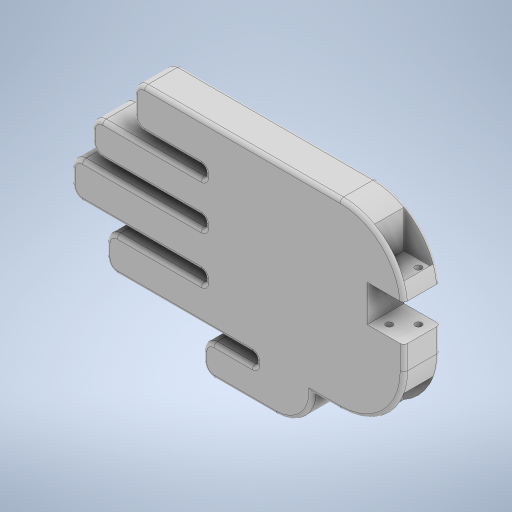
# Autodesk Inventor part: Handv3
Saved by Autodesk Inventor 2024 (Build 280153000, 153)
## iProperties
Created: 2024-02-01
Part Number: Handv3
Material: Generic
Document SubType Name: Modeling
Designer: Irwin
Density: 1 g/cm^3
Appearance: Default
Author: Irwin
Autodesk Inventor part; units mm, degrees
ref_plane "XY Plane" through (0, 0, 0) normal (0, 0, 1) x (1, 0, 0)
sketch "Sketch1" plane through (0, 0, 0) normal (0, 0, 1) x (1, 0, 0)
  line L0 (0, 0) -> (-95, 0)
  line L1 (-95, 0) -> (-95, 100)
  line L2 (-95, 100) -> (0, 100)
  line L3 (0, 100) -> (0, 0)
  dimension "d0" = 100
  dimension "d1" = 95
  constraints: 8 end point, 2 parallel, 1 horizontal, 1 perpendicular
  measures "d0" distance of L2.end L0.start
  measures "d1" distance of L0.start L0.end
extrude "Extrusion1" add sketch "Sketch1" against normal blind 20
sketch "Sketch2" plane through (-95, 0, 0) normal (-1, 0, 0) x (0, 0, 1)
  circle A0 centre (-10, 10) radius 10
  circle A1 centre (-10, 37) radius 10
  circle A2 centre (-10, 63) radius 10
  circle A3 centre (-10, 90) radius 10
  line L0 (0, 0) -> (-20, 0) projected
  line L1 (0, 100) -> (-20, 100) projected
  line L2 (-20, 0) -> (-20, 100) projected
  line L3 (0, 0) -> (-20, 0)
  line L4 (-20, 0) -> (-20, 25)
  line L5 (-20, 25) -> (0, 25)
  line L6 (0, 25) -> (0, 0)
  line L7 (-20, 25) -> (0, 25)
  line L8 (0, 25) -> (0, 50)
  line L9 (0, 50) -> (-20, 50)
  line L10 (-20, 50) -> (-20, 25)
  line L11 (0, 50) -> (-20, 50)
  line L12 (-20, 50) -> (-20, 75)
  line L13 (-20, 75) -> (0, 75)
  line L14 (0, 75) -> (0, 50)
  line L15 (-20, 75) -> (0, 75)
  line L16 (0, 75) -> (0, 100)
  line L17 (0, 100) -> (-20, 100)
  line L18 (-20, 100) -> (-20, 75)
  point P0 (0, 90)
  point P1 (-20, 90)
  point P2 (-10, 100)
  point P3 (0, 37)
  point P4 (-20, 37)
  point P5 (0, 63)
  point P6 (-20, 63)
  point P7 (0, 10)
  point P8 (-20, 10)
  point P9 (-10, 0)
  dimension "d4" = 20
  dimension "d5" = 20
  dimension "d6" = 20
  dimension "d7" = 20
  dimension "d8" = 10
  dimension "d10" = 27
  dimension "d11" = 27
  constraints: 32 end point, 8 parallel, 4 centre point, 4 horizontal, 4 perpendicular, 3 point on line, 3 vertical alignment, 2 tangent
  measures "d4" diameter of A0
  measures "d5" diameter of A1
  measures "d6" diameter of A2
  measures "d7" diameter of A3
  measures "d8" distance from line of L2 A0.centre
  measures "d10" distance of A3.centre A2.centre
  measures "d11" distance of A0.centre A1.centre
extrude "Extrusion2" add sketch "Sketch2" along normal blind 53 contours L13 L2 A3 L16 | A3 | A3 L1 L16 | L2 L1 A3
extrude "Extrusion3" add sketch "Sketch2" along normal blind 76 contours L9 L2 A2 L14 | A2 | A2 L2 L13 L14
extrude "Extrusion4" add sketch "Sketch2" along normal blind 87 contours L5 L2 A1 L8 | A1 | A1 L2 L9 L8
extrude "Extrusion5" add sketch "Sketch2" along normal blind 68 contours A0 | L6 L0 A0 | A0 L2 L5 L6 | A0 L0 L2
fillet "Fillet1" radius 35 2 edges at (0, 0, -10) (0, 100, -10)
sketch "Sketch14" plane through (0, 0, -20) normal (0, 0, -1) x (-1, 0, 0)
  point P0 (0, 0)
ref_plane "Work Plane3" through (0, 65, 0) normal (0, 1, 0) x (-1, 0, 0)
ref_plane "Work Plane4" through (-70, 0, 0) normal (1, 0, 0) x (0, 1, 0)
sketch "Sketch18" plane through (-70, 0, 0) normal (1, 0, 0) x (0, 1, 0)
  line L0 (0, 0) -> (0, -20) projected
  line L1 (0, 0) -> (-20, 0)
  line L2 (-20, 0) -> (-20, -20)
  line L3 (-20, -20) -> (0, -20)
  line L4 (0, -20) -> (0, 0)
  dimension "d63" = 20
  dimension "d64" = 20
  constraints: 8 end point, 2 parallel, 1 horizontal, 1 perpendicular
  measures "d63" distance of L1.end L2.end
  measures "d64" distance of L2.end L3.end
extrude "Extrusion10" add sketch "Sketch18" against normal blind 40
sketch "Sketch19" plane through (-70, 0, 0) normal (1, 0, 0) x (0, 0, -1)
  line L0 (0, -20) -> (20, -20) projected
  line L1 (0, 0) -> (0, -20) projected
  line L2 (20, -20) -> (20, 0) projected
  line L3 (0, 0) -> (20, 0) projected
revolve "Revolution7" add sketch "Sketch19" angle 90 about axis through (-70, 0, 0) along (0, 0, 1)
sketch "Sketch24" plane through (0, 0, 0) normal (0, 0, 1) x (1, 0, 0)
  line L0 (0, 68) -> (-20, 68)
  line L1 (-20, 68) -> (-20, 48)
  line L2 (-20, 48) -> (0, 48)
  line L3 (0, 48) -> (0, 68)
  point P0 (0, 0)
  dimension "d98" = 20
  dimension "d99" = 20
  dimension "d100" = 48
  dimension "d101" = 20
  constraints: 8 end point, 2 parallel, 1 horizontal, 1 perpendicular
  measures "d98" distance of L2.end L1.end
  measures "d99" distance of L1.end L0.end
  measures "d100" distance from line of point (0, 0) L2
  measures "d101" distance from line of point (0, 0) L1
extrude "Extrusion14" cut sketch "Sketch24" against normal blind 20
sketch "Sketch25" plane through (-148, 100, 0) normal (0, 1, 0) x (1, 0, 0)
  line L0 (148, 0) -> (128, 0)
  line L1 (128, 0) -> (128, 20)
  line L2 (128, 20) -> (148, 20)
  line L3 (148, 20) -> (148, 0)
  line L4 (146, 18) -> (130, 18)
  line L5 (130, 18) -> (130, 2)
  line L6 (130, 2) -> (146, 2)
  line L7 (146, 2) -> (146, 18)
  dimension "d104" = 20
  dimension "d105" = 20
  constraints: 16 end point, 4 parallel, 2 perpendicular, 1 horizontal, 3 other
  measures "d104" distance of L1.end L2.end
  measures "d105" distance of L0.end L1.end
extrude "Extrusion15" cut sketch "Sketch25" against normal blind 25 contours L7 L6 L5 L4
sketch "Sketch26" plane through (-35, 0, -20) normal (0, -1, 0) x (1, 0, 0)
  line L0 (35, 20) -> (15, 20)
  line L1 (15, 20) -> (15, 0)
  line L2 (15, 0) -> (35, 0)
  line L3 (35, 0) -> (35, 20)
  line L4 (17, 18) -> (33, 18)
  line L5 (33, 18) -> (33, 2)
  line L6 (33, 2) -> (17, 2)
  line L7 (17, 2) -> (17, 18)
  point P0 (29, 6)
  point P1 (21, 14)
  point P2 (21, 6)
  point P3 (29, 14)
  dimension "d108" = 20
  dimension "d109" = 20
  dimension "d112" = 8
  dimension "d113" = 8
  dimension "d114" = 6
  dimension "d115" = 6
  constraints: 16 end point, 4 parallel, 2 horizontal alignment, 2 perpendicular, 2 vertical alignment, 1 horizontal, 3 other
  measures "d108" distance of L2.end L1.end
  measures "d109" distance of L1.end L0.end
  measures "d112" distance of point (21, 14) point (29, 14)
  measures "d113" distance of point (29, 14) point (29, 6)
  measures "d114" distance from line of L1 point (21, 6)
  measures "d115" distance from line of L0 point (29, 14)
extrude "Extrusion16" cut sketch "Sketch26" against normal blind 40 contours L4 L5 L6 L7
hole "Hole1" at (-14, 0, -6) at (-6, 0, -14) direction (0, 1, 0) diameter 3.6 end through all clearance for "Flat Head Machine Screw" size "M3" standard "Ansi Metric M Profile"
sketch "Sketch27" plane through (0, 0, -20) normal (0, 0, -1) x (-1, 0, 0)
  line L0 (182, 22) -> (109, 22)
  line L1 (109, 22) -> (109, 28)
  line L2 (109, 28) -> (182, 28)
  line L3 (182, 28) -> (182, 22)
  line L4 (182, 48) -> (109, 48)
  line L5 (109, 48) -> (109, 54)
  line L6 (109, 54) -> (182, 54)
  line L7 (182, 54) -> (182, 48)
  line L8 (172, 72) -> (109, 72)
  line L9 (109, 72) -> (109, 78)
  line L10 (109, 78) -> (172, 78)
  line L11 (172, 78) -> (172, 72)
  line L12 (163, -3) -> (81, -3)
  line L13 (81, -3) -> (81, 3)
  line L14 (81, 3) -> (163, 3)
  line L15 (163, 3) -> (163, -3)
  point P0 (0, 0)
  constraints: 32 end point, 8 parallel, 4 horizontal, 4 perpendicular, 1 point on line
extrude "Extrusion17" cut sketch "Sketch27" against normal through all
fillet "Fillet17" radius 6 10 edges at (-110, -20, -10) (-110, -3, -10) (-163, 3, -10) (-163, 22, -10) (-182, 28, -10) (-182, 48, -10) (-171, 54, -10) (-171, 72, -10) (-148, 100, -10) (-148, 78, -10)
fillet "Fillet18" radius 2 8 edges at (-81, -3, -10) (-81, 3, -10) (-109, 22, -10) (-109, 28, -10) (-109, 48, -10) (-109, 54, -10) (-109, 72, -10) (-109, 78, -10)
fillet "Fillet19" radius 2 30 edges at (-148, 89, 0) (-171, 63, 0) (-182, 38, 0) (-163, 12.5, 0) (-120, 3, 0) (-81.5858, 2.4142, 0) (-81, 0, 0) (-110, -11.5, 0) (-87, -20, 0) (-55.8579, -14.1421, 0) (-11.3357, 90.7876, 0) (-88.5, 100, 0) (-148, 89, -20) (-171, 63, -20) (-182, 38, -20) (-163, 12.5, -20) (-120, 3, -20) (-81.5858, 2.4142, -20) (-81, 0, -20) (-110, -11.5, -20) (-87, -20, -20) (-55.8579, -14.1421, -20) (-11.3357, 90.7876, -20) (-88.5, 100, -20) (0, 41.5, -20) (-42.5, 0, -20) (-10.2513, 10.2513, -20) (-42.5, 0, 0) (0, 41.5, 0) (-10.2513, 10.2513, 0)
body "Solid1"
